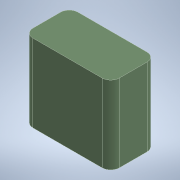
# Autodesk Inventor part: Fix
Saved by Autodesk Inventor 2022 (Build 260153000, 153)
## iProperties
Created: 2023-08-29
Part Number: Fix
Material: Типовые
Document SubType Name: Modeling
Designer: user
Density: 1 g/cm^3
Appearance: По умолчанию
Author: user
## iProperties of the stored document Fix_3DПЕЧАТЬ.ipt
Created: 2023-08-30
Part Number: Fix_3DПЕЧАТЬ
Material: Типовые
Document SubType Name: Modeling
Designer: user
Density: 1 g/cm^3
Appearance: По умолчанию
Author: user
Autodesk Inventor part; units mm, degrees
ref_plane "YZ Plane" through (0, 0, 0) normal (1, 0, 0) x (0, 1, 0)
ref_plane "XZ Plane" through (0, 0, 0) normal (0, 1, 0) x (-1, 0, 0)
ref_plane "XY Plane" through (0, 0, 0) normal (0, 0, 1) x (1, 0, 0)
sketch "Эскиз1" plane through (0, 0, 0) normal (0, 0, 1) x (1, 0, 0)
  line L0 (50, -29) -> (40, -29)
  line L1 (40, -29) -> (40, -20)
  line L2 (40, -20) -> (50, -20)
  line L3 (50, -20) -> (50, -29)
  point P0 (0, 0)
  dimension "d0" = 10
  dimension "d1" = 9
  dimension "d2" = 40
  dimension "d3" = 20
  constraints: 8 end point, 2 parallel, 1 horizontal, 1 perpendicular
  measures "d0" distance of L1.end L2.end
  measures "d1" distance of L0.end L1.end
  measures "d2" distance from line of point (0, 0) L1
  measures "d3" distance from line of point (0, 0) L2
extrude "Выдавливание1" add sketch "Эскиз1" along normal blind 5.2
fillet "Сопряжение1" radius 1 4 edges at (50, -24.5, 5.2) (40, -24.5, 5.2) (50, -24.5, 0) (40, -24.5, 0)
